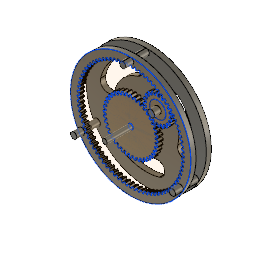
geaarttestv7 (Autodesk Fusion 360 design; units mm, degrees)
description: Spur Gear; Module: 2.025000; Num Teeth: 20; Pressure Angle: 20.000000;
description: Spur Gear; Module: 2.012500; Num Teeth: 40; Pressure Angle: 20.000000;
description: Internal Gear; Module: 2.006300; Num Teeth: 80; Pressure Angle: 20.000000;
Autodesk Fusion 360 part; units mm, degrees
note: some values were not read from the file. Chosen so that the rebuilt part matches the saved one: which face or edge a step refers to. Set by a fixed rule: which sketch regions a step uses.
(part 1 of 7)
sketch "sketch 24727" plane through (0, 0, 0) normal (0, 1, 0) x (1, 0, 0)
  arc A0 (9.2346, -15.5837) -> (8.6942, -15.4391) centre (8.8905, -15.7876) ccw
  spline S0 degree 3 poles (1.6734, -19.8471) (1.7782, -19.3656) (1.7806, -19.0777) (1.7776, -18.982) knots 0 0 0 0 1 1 1 1
  line L0 (3.967, -17.6746) -> (4.1752, -18.6023)
  arc A1 (2.0411, -17.6008) -> (1.6889, -18.0354) centre (2.0872, -17.9981) ccw
  arc A2 (16.6308, -7.1795) -> (16.1086, -7.3802) centre (16.4723, -7.5468) ccw
  arc A3 (20.9592, -7.549) -> (21.3935, -6.2122) centre (0, 0) ccw
  arc A4 (15.4391, -8.6942) -> (16.1086, -7.3802) centre (0, 0) ccw
  spline S1 degree 3 poles (19.3928, -4.5416) (18.9673, -4.2932) (18.6942, -4.2018) (18.6023, -4.1752) knots 0 0 0 0 1 1 1 1
  arc A5 (3.967, -17.6746) -> (3.4977, -17.3701) centre (3.5767, -17.7622) ccw
  arc A6 (-0.7028, -22.2661) -> (0.7028, -22.2661) centre (0, 0) ccw
  arc A7 (18.0354, -1.6889) -> (17.6008, -2.0411) centre (17.9981, -2.0872) ccw
  circle A8 centre (0, 0) radius 12.5
  line L1 (18.0354, -1.6889) -> (18.982, -1.7776)
  arc A9 (7.3802, -16.1086) -> (8.6942, -15.4391) centre (0, 0) ccw
  arc A10 (12.5191, -18.4268) -> (13.6563, -17.6006) centre (0, 0) ccw
  spline S2 degree 3 poles (17.0403, -10.312) (16.7123, -9.9443) (16.4808, -9.773) (16.4016, -9.7193) knots 0 0 0 0 1 1 1 1
  arc A11 (7.3802, -16.1086) -> (7.1795, -16.6308) centre (7.5468, -16.4723) ccw
  spline S3 degree 3 poles (7.7246, -18.3586) (7.6754, -17.8683) (7.5888, -17.5937) (7.5563, -17.5037) knots 0 0 0 0 1 1 1 1
  arc A12 (17.6006, -13.6563) -> (18.4268, -12.5191) centre (0, 0) ccw
  spline S4 degree 3 poles (15.0717, -13.0196) (15.6108, -13.2551) (16.4387, -13.5224) (17.6006, -13.6563) knots 0 0 0 0 1 1 1 1
  arc A13 (15.4391, -8.6942) -> (15.5837, -9.2346) centre (15.7876, -8.8905) ccw
  spline S5 degree 3 poles (21.3935, -6.2122) (20.6023, -5.3509) (19.8994, -4.8382) (19.3928, -4.5416) knots 0 0 0 0 1 1 1 1
  arc A14 (13.5982, -11.9673) -> (13.0396, -11.9968) centre (13.334, -12.2676) ccw
  arc A15 (17.3701, -3.4977) -> (17.6008, -2.0411) centre (0, 0) ccw
  spline S6 degree 3 poles (7.549, -20.9592) (7.7807, -19.8128) (7.7824, -18.9428) (7.7246, -18.3586) knots 0 0 0 0 1 1 1 1
  line L2 (18.6023, -4.1752) -> (17.6746, -3.967)
  arc A16 (17.3701, -3.4977) -> (17.6746, -3.967) centre (17.7622, -3.5767) ccw
  line L3 (1.7776, -18.982) -> (1.6889, -18.0354)
  spline S7 degree 3 poles (0.7028, -22.2661) (1.2774, -21.2475) (1.5478, -20.4206) (1.6734, -19.8471) knots 0 0 0 0 1 1 1 1
  arc A17 (2.0411, -17.6008) -> (3.4977, -17.3701) centre (0, 0) ccw
  line L4 (7.5563, -17.5037) -> (7.1795, -16.6308)
  spline S8 degree 3 poles (13.0197, -15.073) (12.8214, -14.6219) (12.6541, -14.3875) (12.5955, -14.312) knots 0 0 0 0 1 1 1 1
  line L5 (9.2346, -15.5837) -> (9.7193, -16.4016)
  line L6 (16.4016, -9.7193) -> (15.5837, -9.2346)
  line L7 (12.5955, -14.312) -> (11.9673, -13.5982)
  arc A18 (11.9968, -13.0396) -> (11.9673, -13.5982) centre (12.2676, -13.334) ccw
  spline S9 degree 3 poles (13.6563, -17.6006) (13.5224, -16.4387) (13.2551, -15.6108) (13.0197, -15.073) knots 0 0 0 0 1 1 1 1
  spline S10 degree 3 poles (10.3107, -17.0398) (10.7507, -17.4304) (11.4555, -17.9404) (12.5191, -18.4268) knots 0 0 0 0 1 1 1 1
  spline S11 degree 3 poles (9.7193, -16.4016) (9.773, -16.4808) (9.9443, -16.7123) (10.3107, -17.0398) knots 0 0 0 0 1 1 1 1
  arc A19 (11.9968, -13.0396) -> (13.0396, -11.9968) centre (0, 0) ccw
  line L8 (13.5982, -11.9673) -> (14.312, -12.5955)
  spline S12 degree 3 poles (18.3573, -7.725) (18.9428, -7.7824) (19.8128, -7.7807) (20.9592, -7.549) knots 0 0 0 0 1 1 1 1
  spline S13 degree 3 poles (18.4268, -12.5191) (17.9404, -11.4555) (17.4304, -10.7507) (17.0403, -10.312) knots 0 0 0 0 1 1 1 1
  line L9 (16.6308, -7.1795) -> (17.5037, -7.5563)
  spline S14 degree 3 poles (17.5037, -7.5563) (17.5937, -7.5888) (17.8683, -7.6754) (18.3573, -7.725) knots 0 0 0 0 1 1 1 1
  spline S15 degree 3 poles (4.5405, -19.392) (4.8382, -19.8994) (5.3509, -20.6023) (6.2122, -21.3935) knots 0 0 0 0 1 1 1 1
  spline S16 degree 3 poles (14.312, -12.5955) (14.3875, -12.6541) (14.6219, -12.8214) (15.0717, -13.0196) knots 0 0 0 0 1 1 1 1
  arc A20 (6.2122, -21.3935) -> (7.549, -20.9592) centre (0, 0) ccw
  spline S17 degree 3 poles (4.1752, -18.6023) (4.2018, -18.6942) (4.2932, -18.9673) (4.5405, -19.392) knots 0 0 0 0 1 1 1 1
  spline S18 degree 3 poles (-1.6742, -19.846) (-1.5478, -20.4206) (-1.2774, -21.2475) (-0.7028, -22.2661) knots 0 0 0 0 1 1 1 1
  spline S19 degree 3 poles (-1.7776, -18.982) (-1.7806, -19.0777) (-1.7782, -19.3656) (-1.6742, -19.846) knots 0 0 0 0 1 1 1 1
  line L10 (15.5837, 9.2346) -> (16.4016, 9.7193)
  arc A21 (15.5837, 9.2346) -> (15.4391, 8.6942) centre (15.7876, 8.8905) ccw
  spline S20 degree 3 poles (18.3586, 7.7246) (17.8683, 7.6754) (17.5937, 7.5888) (17.5037, 7.5563) knots 0 0 0 0 1 1 1 1
  line L11 (14.312, 12.5955) -> (13.5982, 11.9673)
  spline S21 degree 3 poles (19.8471, 1.6734) (19.3656, 1.7782) (19.0777, 1.7806) (18.982, 1.7776) knots 0 0 0 0 1 1 1 1
  arc A22 (21.3935, 6.2122) -> (20.9592, 7.549) centre (0, 0) ccw
  line L12 (17.5037, 7.5563) -> (16.6308, 7.1795)
  line L13 (11.9673, 13.5982) -> (12.5955, 14.312)
  spline S22 degree 3 poles (15.073, 13.0197) (14.6219, 12.8214) (14.3875, 12.6541) (14.312, 12.5955) knots 0 0 0 0 1 1 1 1
  arc A23 (11.9673, 13.5982) -> (11.9968, 13.0396) centre (12.2676, 13.334) ccw
  arc A24 (13.0396, 11.9968) -> (13.5982, 11.9673) centre (13.334, 12.2676) ccw
  arc A25 (13.0396, 11.9968) -> (11.9968, 13.0396) centre (0, 0) ccw
  spline S23 degree 3 poles (13.0196, 15.0717) (13.2551, 15.6108) (13.5224, 16.4387) (13.6563, 17.6006) knots 0 0 0 0 1 1 1 1
  spline S24 degree 3 poles (18.982, -1.7776) (19.0777, -1.7806) (19.3656, -1.7782) (19.846, -1.6742) knots 0 0 0 0 1 1 1 1
  spline S25 degree 3 poles (12.5955, 14.312) (12.6541, 14.3875) (12.8214, 14.6219) (13.0196, 15.0717) knots 0 0 0 0 1 1 1 1
  arc A26 (17.6746, 3.967) -> (17.3701, 3.4977) centre (17.7622, 3.5767) ccw
  spline S26 degree 3 poles (19.392, 4.5405) (19.8994, 4.8382) (20.6023, 5.3509) (21.3935, 6.2122) knots 0 0 0 0 1 1 1 1
  arc A27 (16.1086, 7.3802) -> (15.4391, 8.6942) centre (0, 0) ccw
  line L14 (18.982, 1.7776) -> (18.0354, 1.6889)
  arc A28 (17.6008, 2.0411) -> (17.3701, 3.4977) centre (0, 0) ccw
  arc A29 (22.2661, -0.7028) -> (22.2661, 0.7028) centre (0, 0) ccw
  spline S27 degree 3 poles (19.846, -1.6742) (20.4206, -1.5478) (21.2475, -1.2774) (22.2661, -0.7028) knots 0 0 0 0 1 1 1 1
  spline S28 degree 3 poles (22.2661, 0.7028) (21.2475, 1.2774) (20.4206, 1.5478) (19.8471, 1.6734) knots 0 0 0 0 1 1 1 1
  arc A30 (17.6008, 2.0411) -> (18.0354, 1.6889) centre (17.9981, 2.0872) ccw
  line L15 (17.6746, 3.967) -> (18.6023, 4.1752)
  spline S29 degree 3 poles (20.9592, 7.549) (19.8128, 7.7807) (18.9428, 7.7824) (18.3586, 7.7246) knots 0 0 0 0 1 1 1 1
  spline S30 degree 3 poles (18.6023, 4.1752) (18.6942, 4.2018) (18.9673, 4.2932) (19.392, 4.5405) knots 0 0 0 0 1 1 1 1
  spline S31 degree 3 poles (16.4016, 9.7193) (16.4808, 9.773) (16.7123, 9.9443) (17.0398, 10.3107) knots 0 0 0 0 1 1 1 1
  arc A31 (18.4268, 12.5191) -> (17.6006, 13.6563) centre (0, 0) ccw
  spline S32 degree 3 poles (17.6006, 13.6563) (16.4387, 13.5224) (15.6108, 13.2551) (15.073, 13.0197) knots 0 0 0 0 1 1 1 1
  spline S33 degree 3 poles (17.0398, 10.3107) (17.4304, 10.7507) (17.9404, 11.4555) (18.4268, 12.5191) knots 0 0 0 0 1 1 1 1
  arc A32 (16.1086, 7.3802) -> (16.6308, 7.1795) centre (16.4723, 7.5468) ccw
  spline S34 degree 3 poles (1.6742, 19.846) (1.5478, 20.4206) (1.2774, 21.2475) (0.7028, 22.2661) knots 0 0 0 0 1 1 1 1
  spline S35 degree 3 poles (1.7776, 18.982) (1.7806, 19.0777) (1.7782, 19.3656) (1.6742, 19.846) knots 0 0 0 0 1 1 1 1
  line L16 (-7.5563, 17.5037) -> (-7.1795, 16.6308)
  spline S36 degree 3 poles (-15.0717, 13.0196) (-15.6108, 13.2551) (-16.4387, 13.5224) (-17.6006, 13.6563) knots 0 0 0 0 1 1 1 1
  arc A33 (-6.2122, 21.3935) -> (-7.549, 20.9592) centre (0, 0) ccw
  arc A34 (-3.967, 17.6746) -> (-3.4977, 17.3701) centre (-3.5767, 17.7622) ccw
  arc A35 (3.4977, 17.3701) -> (3.967, 17.6746) centre (3.5767, 17.7622) ccw
  spline S37 degree 3 poles (-4.5405, 19.392) (-4.8382, 19.8994) (-5.3509, 20.6023) (-6.2122, 21.3935) knots 0 0 0 0 1 1 1 1
  arc A36 (-13.5982, 11.9673) -> (-13.0396, 11.9968) centre (-13.334, 12.2676) ccw
  arc A37 (-15.4391, 8.6942) -> (-15.5837, 9.2346) centre (-15.7876, 8.8905) ccw
  arc A38 (8.6942, 15.4391) -> (7.3802, 16.1086) centre (0, 0) ccw
  spline S38 degree 3 poles (-17.0403, 10.312) (-16.7123, 9.9443) (-16.4808, 9.773) (-16.4016, 9.7193) knots 0 0 0 0 1 1 1 1
  spline S39 degree 3 poles (-13.0197, 15.073) (-12.8214, 14.6219) (-12.6541, 14.3875) (-12.5955, 14.312) knots 0 0 0 0 1 1 1 1
  spline S40 degree 3 poles (-1.6734, 19.8471) (-1.7782, 19.3656) (-1.7806, 19.0777) (-1.7776, 18.982) knots 0 0 0 0 1 1 1 1
  spline S41 degree 3 poles (-9.7193, 16.4016) (-9.773, 16.4808) (-9.9443, 16.7123) (-10.3107, 17.0398) knots 0 0 0 0 1 1 1 1
  spline S42 degree 3 poles (-14.312, 12.5955) (-14.3875, 12.6541) (-14.6219, 12.8214) (-15.0717, 13.0196) knots 0 0 0 0 1 1 1 1
  spline S43 degree 3 poles (-18.4268, 12.5191) (-17.9404, 11.4555) (-17.4304, 10.7507) (-17.0403, 10.312) knots 0 0 0 0 1 1 1 1
  line L17 (9.7193, 16.4016) -> (9.2346, 15.5837)
  line L18 (-12.5955, 14.312) -> (-11.9673, 13.5982)
  arc A39 (-2.0411, 17.6008) -> (-1.6889, 18.0354) centre (-2.0872, 17.9981) ccw
  arc A40 (1.6889, 18.0354) -> (2.0411, 17.6008) centre (2.0872, 17.9981) ccw
  spline S44 degree 3 poles (-7.7246, 18.3586) (-7.6754, 17.8683) (-7.5888, 17.5937) (-7.5563, 17.5037) knots 0 0 0 0 1 1 1 1
  spline S45 degree 3 poles (-4.1752, 18.6023) (-4.2018, 18.6942) (-4.2932, 18.9673) (-4.5405, 19.392) knots 0 0 0 0 1 1 1 1
  arc A41 (7.549, 20.9592) -> (6.2122, 21.3935) centre (0, 0) ccw
  arc A42 (13.6563, 17.6006) -> (12.5191, 18.4268) centre (0, 0) ccw
  arc A43 (8.6942, 15.4391) -> (9.2346, 15.5837) centre (8.8905, 15.7876) ccw
  arc A44 (3.4977, 17.3701) -> (2.0411, 17.6008) centre (0, 0) ccw
  spline S46 degree 3 poles (-7.549, 20.9592) (-7.7807, 19.8128) (-7.7824, 18.9428) (-7.7246, 18.3586) knots 0 0 0 0 1 1 1 1
  spline S47 degree 3 poles (10.312, 17.0403) (9.9443, 16.7123) (9.773, 16.4808) (9.7193, 16.4016) knots 0 0 0 0 1 1 1 1
  arc A45 (-9.2346, 15.5837) -> (-8.6942, 15.4391) centre (-8.8905, 15.7876) ccw
  spline S48 degree 3 poles (6.2122, 21.3935) (5.3509, 20.6023) (4.8382, 19.8994) (4.5416, 19.3928) knots 0 0 0 0 1 1 1 1
  line L19 (4.1752, 18.6023) -> (3.967, 17.6746)
  spline S49 degree 3 poles (12.5191, 18.4268) (11.4555, 17.9404) (10.7507, 17.4304) (10.312, 17.0403) knots 0 0 0 0 1 1 1 1
  spline S50 degree 3 poles (-0.7028, 22.2661) (-1.2774, 21.2475) (-1.5478, 20.4206) (-1.6734, 19.8471) knots 0 0 0 0 1 1 1 1
  line L20 (-3.967, 17.6746) -> (-4.1752, 18.6023)
  arc A46 (-7.3802, 16.1086) -> (-7.1795, 16.6308) centre (-7.5468, 16.4723) ccw
  arc A47 (-12.5191, 18.4268) -> (-13.6563, 17.6006) centre (0, 0) ccw
  spline S51 degree 3 poles (7.5563, 17.5037) (7.5888, 17.5937) (7.6754, 17.8683) (7.725, 18.3573) knots 0 0 0 0 1 1 1 1
  line L21 (-1.7776, 18.982) -> (-1.6889, 18.0354)
  spline S52 degree 3 poles (-10.3107, 17.0398) (-10.7507, 17.4304) (-11.4555, 17.9404) (-12.5191, 18.4268) knots 0 0 0 0 1 1 1 1
  arc A48 (7.1795, 16.6308) -> (7.3802, 16.1086) centre (7.5468, 16.4723) ccw
  arc A49 (-2.0411, 17.6008) -> (-3.4977, 17.3701) centre (0, 0) ccw
  line L22 (-9.2346, 15.5837) -> (-9.7193, 16.4016)
  spline S53 degree 3 poles (4.5416, 19.3928) (4.2932, 18.9673) (4.2018, 18.6942) (4.1752, 18.6023) knots 0 0 0 0 1 1 1 1
  spline S54 degree 3 poles (-13.6563, 17.6006) (-13.5224, 16.4387) (-13.2551, 15.6108) (-13.0197, 15.073) knots 0 0 0 0 1 1 1 1
  spline S55 degree 3 poles (7.725, 18.3573) (7.7824, 18.9428) (7.7807, 19.8128) (7.549, 20.9592) knots 0 0 0 0 1 1 1 1
  line L23 (7.1795, 16.6308) -> (7.5563, 17.5037)
  arc A50 (0.7028, 22.2661) -> (-0.7028, 22.2661) centre (0, 0) ccw
  arc A51 (-17.6006, 13.6563) -> (-18.4268, 12.5191) centre (0, 0) ccw
  arc A52 (-11.9968, 13.0396) -> (-11.9673, 13.5982) centre (-12.2676, 13.334) ccw
  line L24 (-13.5982, 11.9673) -> (-14.312, 12.5955)
  arc A53 (-7.3802, 16.1086) -> (-8.6942, 15.4391) centre (0, 0) ccw
  arc A54 (-11.9968, 13.0396) -> (-13.0396, 11.9968) centre (0, 0) ccw
  line L25 (1.6889, 18.0354) -> (1.7776, 18.982)
  arc A55 (-15.4391, 8.6942) -> (-16.1086, 7.3802) centre (0, 0) ccw
  line L26 (-17.5037, -7.5563) -> (-16.6308, -7.1795)
  line L27 (-9.7193, -16.4016) -> (-9.2346, -15.5837)
  arc A56 (-8.6942, -15.4391) -> (-9.2346, -15.5837) centre (-8.8905, -15.7876) ccw
  spline S56 degree 3 poles (-17.0398, -10.3107) (-17.4304, -10.7507) (-17.9404, -11.4555) (-18.4268, -12.5191) knots 0 0 0 0 1 1 1 1
  spline S57 degree 3 poles (-6.2122, -21.3935) (-5.3509, -20.6023) (-4.8382, -19.8994) (-4.5416, -19.3928) knots 0 0 0 0 1 1 1 1
  line L28 (-1.6889, -18.0354) -> (-1.7776, -18.982)
  arc A57 (-17.3701, 3.4977) -> (-17.6008, 2.0411) centre (0, 0) ccw
  line L29 (-18.982, -1.7776) -> (-18.0354, -1.6889)
  spline S58 degree 3 poles (-18.3573, 7.725) (-18.9428, 7.7824) (-19.8128, 7.7807) (-20.9592, 7.549) knots 0 0 0 0 1 1 1 1
  arc A58 (-16.6308, 7.1795) -> (-16.1086, 7.3802) centre (-16.4723, 7.5468) ccw
  spline S59 degree 3 poles (-18.982, 1.7776) (-19.0777, 1.7806) (-19.3656, 1.7782) (-19.846, 1.6742) knots 0 0 0 0 1 1 1 1
  spline S60 degree 3 poles (-13.0196, -15.0717) (-13.2551, -15.6108) (-13.5224, -16.4387) (-13.6563, -17.6006) knots 0 0 0 0 1 1 1 1
  spline S61 degree 3 poles (-17.5037, 7.5563) (-17.5937, 7.5888) (-17.8683, 7.6754) (-18.3573, 7.725) knots 0 0 0 0 1 1 1 1
  arc A59 (-17.6746, -3.967) -> (-17.3701, -3.4977) centre (-17.7622, -3.5767) ccw
  spline S62 degree 3 poles (-20.9592, -7.549) (-19.8128, -7.7807) (-18.9428, -7.7824) (-18.3586, -7.7246) knots 0 0 0 0 1 1 1 1
  line L30 (-16.4016, 9.7193) -> (-15.5837, 9.2346)
  line L31 (-16.6308, 7.1795) -> (-17.5037, 7.5563)
  arc A60 (-17.6008, -2.0411) -> (-18.0354, -1.6889) centre (-17.9981, -2.0872) ccw
  line L32 (-18.6023, 4.1752) -> (-17.6746, 3.967)
  arc A61 (-16.1086, -7.3802) -> (-16.6308, -7.1795) centre (-16.4723, -7.5468) ccw
  line L33 (-15.5837, -9.2346) -> (-16.4016, -9.7193)
  spline S63 degree 3 poles (-19.3928, 4.5416) (-18.9673, 4.2932) (-18.6942, 4.2018) (-18.6023, 4.1752) knots 0 0 0 0 1 1 1 1
  arc A62 (-18.4268, -12.5191) -> (-17.6006, -13.6563) centre (0, 0) ccw
  spline S64 degree 3 poles (-18.3586, -7.7246) (-17.8683, -7.6754) (-17.5937, -7.5888) (-17.5037, -7.5563) knots 0 0 0 0 1 1 1 1
  arc A63 (-13.0396, -11.9968) -> (-11.9968, -13.0396) centre (0, 0) ccw
  line L34 (-11.9673, -13.5982) -> (-12.5955, -14.312)
  arc A64 (-22.2661, 0.7028) -> (-22.2661, -0.7028) centre (0, 0) ccw
  spline S65 degree 3 poles (-17.6006, -13.6563) (-16.4387, -13.5224) (-15.6108, -13.2551) (-15.073, -13.0197) knots 0 0 0 0 1 1 1 1
  spline S66 degree 3 poles (-15.073, -13.0197) (-14.6219, -12.8214) (-14.3875, -12.6541) (-14.312, -12.5955) knots 0 0 0 0 1 1 1 1
  arc A65 (-13.0396, -11.9968) -> (-13.5982, -11.9673) centre (-13.334, -12.2676) ccw
  spline S67 degree 3 poles (-16.4016, -9.7193) (-16.4808, -9.773) (-16.7123, -9.9443) (-17.0398, -10.3107) knots 0 0 0 0 1 1 1 1
  arc A66 (-13.6563, -17.6006) -> (-12.5191, -18.4268) centre (0, 0) ccw
  spline S68 degree 3 poles (-18.6023, -4.1752) (-18.6942, -4.2018) (-18.9673, -4.2932) (-19.392, -4.5405) knots 0 0 0 0 1 1 1 1
  spline S69 degree 3 poles (-22.2661, -0.7028) (-21.2475, -1.2774) (-20.4206, -1.5478) (-19.8471, -1.6734) knots 0 0 0 0 1 1 1 1
  arc A67 (-18.0354, 1.6889) -> (-17.6008, 2.0411) centre (-17.9981, 2.0872) ccw
  arc A68 (-17.3701, 3.4977) -> (-17.6746, 3.967) centre (-17.7622, 3.5767) ccw
  spline S70 degree 3 poles (-21.3935, 6.2122) (-20.6023, 5.3509) (-19.8994, 4.8382) (-19.3928, 4.5416) knots 0 0 0 0 1 1 1 1
  spline S71 degree 3 poles (-19.392, -4.5405) (-19.8994, -4.8382) (-20.6023, -5.3509) (-21.3935, -6.2122) knots 0 0 0 0 1 1 1 1
  arc A69 (-21.3935, -6.2122) -> (-20.9592, -7.549) centre (0, 0) ccw
  arc A70 (-15.5837, -9.2346) -> (-15.4391, -8.6942) centre (-15.7876, -8.8905) ccw
  arc A71 (-17.6008, -2.0411) -> (-17.3701, -3.4977) centre (0, 0) ccw
  line L35 (-17.6746, -3.967) -> (-18.6023, -4.1752)
  arc A72 (-11.9673, -13.5982) -> (-11.9968, -13.0396) centre (-12.2676, -13.334) ccw
  spline S72 degree 3 poles (-10.312, -17.0403) (-9.9443, -16.7123) (-9.773, -16.4808) (-9.7193, -16.4016) knots 0 0 0 0 1 1 1 1
  arc A73 (-20.9592, 7.549) -> (-21.3935, 6.2122) centre (0, 0) ccw
  arc A74 (-8.6942, -15.4391) -> (-7.3802, -16.1086) centre (0, 0) ccw
  spline S73 degree 3 poles (-12.5191, -18.4268) (-11.4555, -17.9404) (-10.7507, -17.4304) (-10.312, -17.0403) knots 0 0 0 0 1 1 1 1
  spline S74 degree 3 poles (-12.5955, -14.312) (-12.6541, -14.3875) (-12.8214, -14.6219) (-13.0196, -15.0717) knots 0 0 0 0 1 1 1 1
  spline S75 degree 3 poles (-19.846, 1.6742) (-20.4206, 1.5478) (-21.2475, 1.2774) (-22.2661, 0.7028) knots 0 0 0 0 1 1 1 1
  line L36 (-7.1795, -16.6308) -> (-7.5563, -17.5037)
  spline S76 degree 3 poles (-7.5563, -17.5037) (-7.5888, -17.5937) (-7.6754, -17.8683) (-7.725, -18.3573) knots 0 0 0 0 1 1 1 1
  arc A75 (-7.1795, -16.6308) -> (-7.3802, -16.1086) centre (-7.5468, -16.4723) ccw
  spline S77 degree 3 poles (-7.725, -18.3573) (-7.7824, -18.9428) (-7.7807, -19.8128) (-7.549, -20.9592) knots 0 0 0 0 1 1 1 1
  arc A76 (-16.1086, -7.3802) -> (-15.4391, -8.6942) centre (0, 0) ccw
  arc A77 (-7.549, -20.9592) -> (-6.2122, -21.3935) centre (0, 0) ccw
  line L37 (-18.0354, 1.6889) -> (-18.982, 1.7776)
  spline S78 degree 3 poles (-19.8471, -1.6734) (-19.3656, -1.7782) (-19.0777, -1.7806) (-18.982, -1.7776) knots 0 0 0 0 1 1 1 1
  line L38 (-14.312, -12.5955) -> (-13.5982, -11.9673)
  line L39 (-4.1752, -18.6023) -> (-3.967, -17.6746)
  arc A78 (-1.6889, -18.0354) -> (-2.0411, -17.6008) centre (-2.0872, -17.9981) ccw
  arc A79 (-3.4977, -17.3701) -> (-2.0411, -17.6008) centre (0, 0) ccw
  arc A80 (-3.4977, -17.3701) -> (-3.967, -17.6746) centre (-3.5767, -17.7622) ccw
  spline S79 degree 3 poles (-4.5416, -19.3928) (-4.2932, -18.9673) (-4.2018, -18.6942) (-4.1752, -18.6023) knots 0 0 0 0 1 1 1 1
extrude "Extrude1" add sketch "sketch 24727" along normal blind 8 makes body 1 in component "Spur Gear (20 teeth)"
sketch "Sketch1" plane through (0, 0, 0) normal (0, 1, 0) x (1, 0, 0) in component "Spur Gear (20 teeth)"
  circle A0 centre (0, 0) radius 20.25 construction
sketch "sketch 26269" plane through (0, 0, 0) normal (0, 1, 0) x (1, 0, 0)
  spline S0 degree 3 poles (-13.6938, -35.5383) (-13.7432, -35.732) (-13.808, -36.0399) (-13.8582, -36.4722) knots 0 0 0 0 1 1 1 1
  spline S1 degree 3 poles (-24.2197, -34.6367) (-22.8543, -33.8927) (-21.9375, -33.1795) (-21.3609, -32.6493) knots 0 0 0 0 1 1 1 1
  spline S2 degree 3 poles (-18.5031, -37.999) (-17.271, -37.0506) (-16.477, -36.2028) (-15.9905, -35.5889) knots 0 0 0 0 1 1 1 1
  arc A0 (-20.1803, -31.8848) -> (-19.2479, -32.4562) centre (0, 0) ccw
  arc A1 (-14.944, -34.6491) -> (-13.9336, -35.0676) centre (0, 0) ccw
  arc A2 (-14.944, -34.6491) -> (-15.4464, -34.8123) centre (-15.1024, -35.0164) ccw
  spline S3 degree 3 poles (-15.9905, -35.5889) (-15.7204, -35.2478) (-15.5484, -34.9843) (-15.4464, -34.8123) knots 0 0 0 0 1 1 1 1
  arc A3 (-13.6938, -35.5383) -> (-13.9336, -35.0676) centre (-14.0813, -35.4393) ccw
  arc A4 (-13.7857, -39.953) -> (-12.331, -40.4257) centre (0, 0) ccw
  spline S4 degree 3 poles (-19.0846, -32.9586) (-19.1638, -33.1422) (-19.2759, -33.4362) (-19.3931, -33.8552) knots 0 0 0 0 1 1 1 1
  spline S5 degree 3 poles (-12.331, -40.4257) (-11.2623, -39.2962) (-10.6107, -38.3346) (-10.2263, -37.6523) knots 0 0 0 0 1 1 1 1
  spline S6 degree 3 poles (-21.3609, -32.6493) (-21.0408, -32.3546) (-20.8297, -32.1213) (-20.7021, -31.9674) knots 0 0 0 0 1 1 1 1
  arc A5 (-20.1803, -31.8848) -> (-20.7021, -31.9674) centre (-20.3942, -32.2228) ccw
  arc A6 (-19.866, -37.3046) -> (-18.5031, -37.999) centre (0, 0) ccw
  spline S7 degree 3 poles (-19.3931, -33.8552) (-19.6037, -34.6096) (-19.823, -35.7503) (-19.866, -37.3046) knots 0 0 0 0 1 1 1 1
  spline S8 degree 3 poles (-7.9658, -37.243) (-7.9843, -37.442) (-8.0001, -37.7562) (-7.9821, -38.191) knots 0 0 0 0 1 1 1 1
  arc A7 (-7.9658, -37.243) -> (-8.2763, -36.8156) centre (-8.364, -37.2058) ccw
  arc A8 (-9.3397, -36.5603) -> (-8.2763, -36.8156) centre (0, 0) ccw
  arc A9 (-9.3397, -36.5603) -> (-9.8104, -36.8001) centre (-9.4387, -36.9478) ccw
  spline S9 degree 3 poles (-13.8582, -36.4722) (-13.9482, -37.2502) (-13.9863, -38.4112) (-13.7857, -39.953) knots 0 0 0 0 1 1 1 1
  spline S10 degree 3 poles (-10.2263, -37.6523) (-10.0128, -37.273) (-9.8842, -36.9859) (-9.8104, -36.8001) knots 0 0 0 0 1 1 1 1
  spline S11 degree 3 poles (-5.8552, -41.857) (-4.9764, -40.5743) (-4.4833, -39.5225) (-4.2102, -38.7884) knots 0 0 0 0 1 1 1 1
  arc A10 (-3.5054, -37.5712) -> (-2.4152, -37.657) centre (0, 0) ccw
  arc A11 (-3.5054, -37.5712) -> (-3.9328, -37.8817) centre (-3.5426, -37.9695) ccw
  spline S12 degree 3 poles (-1.9094, -38.9695) (-1.7546, -39.7373) (-1.4321, -40.8532) (-0.7648, -42.2576) knots 0 0 0 0 1 1 1 1
  arc A12 (-0.7648, -42.2576) -> (0.7648, -42.2576) centre (0, 0) ccw
  spline S13 degree 3 poles (-4.2102, -38.7884) (-4.0588, -38.3805) (-3.9767, -38.0767) (-3.9328, -37.8817) knots 0 0 0 0 1 1 1 1
  arc A13 (-7.3659, -41.6177) -> (-5.8552, -41.857) centre (0, 0) ccw
  spline S14 degree 3 poles (-7.9821, -38.191) (-7.9493, -38.9736) (-7.8053, -40.1262) (-7.3659, -41.6177) knots 0 0 0 0 1 1 1 1
  spline S15 degree 3 poles (4.2102, -38.7884) (4.4833, -39.5225) (4.9764, -40.5743) (5.8552, -41.857) knots 0 0 0 0 1 1 1 1
  spline S16 degree 3 poles (0.7648, -42.2576) (1.4321, -40.8532) (1.7546, -39.7373) (1.9094, -38.9695) knots 0 0 0 0 1 1 1 1
  spline S17 degree 3 poles (1.9094, -38.9695) (1.9952, -38.5429) (2.0288, -38.23) (2.0416, -38.0306) knots 0 0 0 0 1 1 1 1
  spline S18 degree 3 poles (3.9328, -37.8817) (3.9767, -38.0767) (4.0588, -38.3805) (4.2102, -38.7884) knots 0 0 0 0 1 1 1 1
  spline S19 degree 3 poles (-2.0416, -38.0306) (-2.0288, -38.23) (-1.9952, -38.5429) (-1.9094, -38.9695) knots 0 0 0 0 1 1 1 1
  arc A14 (-2.0416, -38.0306) -> (-2.4152, -37.657) centre (-2.4408, -38.0562) ccw
  arc A15 (2.4152, -37.657) -> (2.0416, -38.0306) centre (2.4408, -38.0562) ccw
  arc A16 (2.4152, -37.657) -> (3.5054, -37.5712) centre (0, 0) ccw
  arc A17 (3.9328, -37.8817) -> (3.5054, -37.5712) centre (3.5426, -37.9695) ccw
  arc A18 (5.8552, -41.857) -> (7.3659, -41.6177) centre (0, 0) ccw
  circle A19 centre (0, 0) radius 3.85
  arc A20 (31.8848, -20.1803) -> (32.4562, -19.2479) centre (0, 0) ccw
  arc A21 (37.5712, -3.5054) -> (37.8817, -3.9328) centre (37.9695, -3.5426) ccw
  spline S20 degree 3 poles (41.857, -5.8552) (40.5743, -4.9764) (39.5225, -4.4833) (38.7884, -4.2102) knots 0 0 0 0 1 1 1 1
  arc A22 (37.5712, -3.5054) -> (37.657, -2.4152) centre (0, 0) ccw
  spline S21 degree 3 poles (38.7884, -4.2102) (38.3805, -4.0588) (38.0767, -3.9767) (37.8817, -3.9328) knots 0 0 0 0 1 1 1 1
  spline S22 degree 3 poles (32.6493, -21.3609) (32.3546, -21.0408) (32.1213, -20.8297) (31.9674, -20.7021) knots 0 0 0 0 1 1 1 1
  arc A23 (31.8848, -20.1803) -> (31.9674, -20.7021) centre (32.2228, -20.3942) ccw
  spline S23 degree 3 poles (34.6367, -24.2197) (33.8927, -22.8543) (33.1795, -21.9375) (32.6493, -21.3609) knots 0 0 0 0 1 1 1 1
  arc A24 (37.3046, -19.866) -> (37.999, -18.5031) centre (0, 0) ccw
  arc A25 (34.6491, -14.944) -> (35.0676, -13.9336) centre (0, 0) ccw
  arc A26 (32.9586, -19.0846) -> (32.4562, -19.2479) centre (32.8002, -19.4519) ccw
  spline S24 degree 3 poles (32.9586, -19.0846) (33.1422, -19.1638) (33.4362, -19.2759) (33.8552, -19.3931) knots 0 0 0 0 1 1 1 1
  spline S25 degree 3 poles (33.8552, -19.3931) (34.6096, -19.6037) (35.7503, -19.823) (37.3046, -19.866) knots 0 0 0 0 1 1 1 1
  spline S26 degree 3 poles (37.999, -18.5031) (37.0506, -17.271) (36.2028, -16.477) (35.5889, -15.9905) knots 0 0 0 0 1 1 1 1
  arc A27 (34.6491, -14.944) -> (34.8123, -15.4464) centre (35.0164, -15.1024) ccw
  arc A28 (36.5603, -9.3397) -> (36.8001, -9.8104) centre (36.9478, -9.4387) ccw
  spline S27 degree 3 poles (35.5889, -15.9905) (35.2478, -15.7204) (34.9843, -15.5484) (34.8123, -15.4464) knots 0 0 0 0 1 1 1 1
  spline S28 degree 3 poles (35.5383, -13.6938) (35.732, -13.7432) (36.0399, -13.808) (36.4722, -13.8582) knots 0 0 0 0 1 1 1 1
  arc A29 (37.243, -7.9658) -> (36.8156, -8.2763) centre (37.2058, -8.364) ccw
  spline S29 degree 3 poles (36.4722, -13.8582) (37.2502, -13.9482) (38.4112, -13.9863) (39.953, -13.7857) knots 0 0 0 0 1 1 1 1
  arc A30 (39.953, -13.7857) -> (40.4257, -12.331) centre (0, 0) ccw
  arc A31 (36.5603, -9.3397) -> (36.8156, -8.2763) centre (0, 0) ccw
  spline S30 degree 3 poles (37.6523, -10.2263) (37.273, -10.0128) (36.9859, -9.8842) (36.8001, -9.8104) knots 0 0 0 0 1 1 1 1
  arc A32 (35.5383, -13.6938) -> (35.0676, -13.9336) centre (35.4393, -14.0813) ccw
  spline S31 degree 3 poles (40.4257, -12.331) (39.2962, -11.2623) (38.3346, -10.6107) (37.6523, -10.2263) knots 0 0 0 0 1 1 1 1
  spline S32 degree 3 poles (37.243, -7.9658) (37.442, -7.9843) (37.7562, -8.0001) (38.191, -7.9821) knots 0 0 0 0 1 1 1 1
  spline S33 degree 3 poles (-38.0306, 2.0416) (-38.23, 2.0288) (-38.5429, 1.9952) (-38.9695, 1.9094) knots 0 0 0 0 1 1 1 1
  arc A33 (-37.5712, 3.5054) -> (-37.8817, 3.9328) centre (-37.9695, 3.5426) ccw
  arc A34 (-37.5712, 3.5054) -> (-37.657, 2.4152) centre (0, 0) ccw
  arc A35 (41.6177, -7.3659) -> (41.857, -5.8552) centre (0, 0) ccw
  spline S34 degree 3 poles (38.191, -7.9821) (38.9736, -7.9493) (40.1262, -7.8053) (41.6177, -7.3659) knots 0 0 0 0 1 1 1 1
  arc A36 (-38.0306, 2.0416) -> (-37.657, 2.4152) centre (-38.0562, 2.4408) ccw
  spline S35 degree 3 poles (-38.7884, 4.2102) (-38.3805, 4.0588) (-38.0767, 3.9767) (-37.8817, 3.9328) knots 0 0 0 0 1 1 1 1
  spline S36 degree 3 poles (-38.9695, -1.9094) (-38.5429, -1.9952) (-38.23, -2.0288) (-38.0306, -2.0416) knots 0 0 0 0 1 1 1 1
  arc A37 (-37.657, -2.4152) -> (-38.0306, -2.0416) centre (-38.0562, -2.4408) ccw
  arc A38 (-42.2576, 0.7648) -> (-42.2576, -0.7648) centre (0, 0) ccw
  arc A39 (-37.657, -2.4152) -> (-37.5712, -3.5054) centre (0, 0) ccw
  arc A40 (-37.8817, -3.9328) -> (-37.5712, -3.5054) centre (-37.9695, -3.5426) ccw
  spline S37 degree 3 poles (-38.9695, 1.9094) (-39.7373, 1.7546) (-40.8532, 1.4321) (-42.2576, 0.7648) knots 0 0 0 0 1 1 1 1
  spline S38 degree 3 poles (-42.2576, -0.7648) (-40.8532, -1.4321) (-39.7373, -1.7546) (-38.9695, -1.9094) knots 0 0 0 0 1 1 1 1
  spline S39 degree 3 poles (-37.8817, -3.9328) (-38.0767, -3.9767) (-38.3805, -4.0588) (-38.7884, -4.2102) knots 0 0 0 0 1 1 1 1
  spline S40 degree 3 poles (-38.7884, -4.2102) (-39.5225, -4.4833) (-40.5743, -4.9764) (-41.857, -5.8552) knots 0 0 0 0 1 1 1 1
  arc A41 (-41.857, -5.8552) -> (-41.6177, -7.3659) centre (0, 0) ccw
  spline S41 degree 3 poles (-38.191, -7.9821) (-37.7562, -8.0001) (-37.442, -7.9843) (-37.243, -7.9658) knots 0 0 0 0 1 1 1 1
  arc A42 (-36.8001, -9.8104) -> (-36.5603, -9.3397) centre (-36.9478, -9.4387) ccw
  arc A43 (-36.8156, -8.2763) -> (-37.243, -7.9658) centre (-37.2058, -8.364) ccw
  arc A44 (-36.8156, -8.2763) -> (-36.5603, -9.3397) centre (0, 0) ccw
  spline S42 degree 3 poles (-41.6177, -7.3659) (-40.1262, -7.8053) (-38.9736, -7.9493) (-38.191, -7.9821) knots 0 0 0 0 1 1 1 1
  arc A45 (-40.4257, -12.331) -> (-39.953, -13.7857) centre (0, 0) ccw
  spline S43 degree 3 poles (-36.8001, -9.8104) (-36.9859, -9.8842) (-37.273, -10.0128) (-37.6523, -10.2263) knots 0 0 0 0 1 1 1 1
  spline S44 degree 3 poles (-36.4722, -13.8582) (-36.0399, -13.808) (-35.732, -13.7432) (-35.5383, -13.6938) knots 0 0 0 0 1 1 1 1
  arc A46 (-35.0676, -13.9336) -> (-35.5383, -13.6938) centre (-35.4393, -14.0813) ccw
  arc A47 (-34.8123, -15.4464) -> (-34.6491, -14.944) centre (-35.0164, -15.1024) ccw
  spline S45 degree 3 poles (-39.953, -13.7857) (-38.4112, -13.9863) (-37.2502, -13.9482) (-36.4722, -13.8582) knots 0 0 0 0 1 1 1 1
  spline S46 degree 3 poles (-37.6523, -10.2263) (-38.3346, -10.6107) (-39.2962, -11.2623) (-40.4257, -12.331) knots 0 0 0 0 1 1 1 1
  arc A48 (-32.4562, -19.2479) -> (-31.8848, -20.1803) centre (0, 0) ccw
  arc A49 (-31.9674, -20.7021) -> (-31.8848, -20.1803) centre (-32.2228, -20.3942) ccw
  spline S47 degree 3 poles (-35.5889, -15.9905) (-36.2028, -16.477) (-37.0506, -17.271) (-37.999, -18.5031) knots 0 0 0 0 1 1 1 1
  arc A50 (-35.0676, -13.9336) -> (-34.6491, -14.944) centre (0, 0) ccw
  spline S48 degree 3 poles (-37.3046, -19.866) (-35.7503, -19.823) (-34.6096, -19.6037) (-33.8552, -19.3931) knots 0 0 0 0 1 1 1 1
  arc A51 (-32.4562, -19.2479) -> (-32.9586, -19.0846) centre (-32.8002, -19.4519) ccw
  arc A52 (-34.6367, -24.2197) -> (-33.7376, -25.4571) centre (0, 0) ccw
  spline S49 degree 3 poles (-34.8123, -15.4464) (-34.9843, -15.5484) (-35.2478, -15.7204) (-35.5889, -15.9905) knots 0 0 0 0 1 1 1 1
  spline S50 degree 3 poles (-32.6493, -21.3609) (-33.1795, -21.9375) (-33.8927, -22.8543) (-34.6367, -24.2197) knots 0 0 0 0 1 1 1 1
  spline S51 degree 3 poles (-33.8552, -19.3931) (-33.4362, -19.2759) (-33.1422, -19.1638) (-32.9586, -19.0846) knots 0 0 0 0 1 1 1 1
  spline S52 degree 3 poles (-33.7376, -25.4571) (-32.2092, -25.1715) (-31.1168, -24.7765) (-30.4047, -24.4505) knots 0 0 0 0 1 1 1 1
  spline S53 degree 3 poles (-28.3353, -25.448) (-28.4673, -25.5981) (-28.6648, -25.8431) (-28.9058, -26.2054) knots 0 0 0 0 1 1 1 1
  arc A53 (-37.999, -18.5031) -> (-37.3046, -19.866) centre (0, 0) ccw
  arc A54 (-29.0455, -24.0882) -> (-28.3353, -24.9197) centre (0, 0) ccw
  spline S54 degree 3 poles (-31.9674, -20.7021) (-32.1213, -20.8297) (-32.3546, -21.0408) (-32.6493, -21.3609) knots 0 0 0 0 1 1 1 1
  spline S55 degree 3 poles (-30.4047, -24.4505) (-30.0091, -24.2691) (-29.7363, -24.1124) (-29.5673, -24.0055) knots 0 0 0 0 1 1 1 1
  arc A55 (-28.3353, -25.448) -> (-28.3353, -24.9197) centre (-28.6357, -25.1839) ccw
  arc A56 (-30.4214, -29.3399) -> (-29.3399, -30.4214) centre (0, 0) ccw
  spline S56 degree 3 poles (-29.3399, -30.4214) (-27.8749, -29.9002) (-26.8578, -29.3392) (-26.2054, -28.9058) knots 0 0 0 0 1 1 1 1
  spline S57 degree 3 poles (-28.9058, -26.2054) (-29.3392, -26.8578) (-29.9002, -27.8749) (-30.4214, -29.3399) knots 0 0 0 0 1 1 1 1
  spline S58 degree 3 poles (-24.4505, -30.4047) (-24.7765, -31.1168) (-25.1715, -32.2092) (-25.4571, -33.7376) knots 0 0 0 0 1 1 1 1
  arc A57 (-25.4571, -33.7376) -> (-24.2197, -34.6367) centre (0, 0) ccw
  arc A58 (-19.0846, -32.9586) -> (-19.2479, -32.4562) centre (-19.4519, -32.8002) ccw
  arc A59 (-29.0455, -24.0882) -> (-29.5673, -24.0055) centre (-29.3534, -24.3435) ccw
  arc A60 (-24.9197, -28.3353) -> (-24.0882, -29.0455) centre (0, 0) ccw
  spline S59 degree 3 poles (-24.0055, -29.5673) (-24.1124, -29.7363) (-24.2691, -30.0091) (-24.4505, -30.4047) knots 0 0 0 0 1 1 1 1
  spline S60 degree 3 poles (-26.2054, -28.9058) (-25.8431, -28.6648) (-25.5981, -28.4673) (-25.448, -28.3353) knots 0 0 0 0 1 1 1 1
  arc A61 (-24.9197, -28.3353) -> (-25.448, -28.3353) centre (-25.1839, -28.6357) ccw
  arc A62 (-24.0055, -29.5673) -> (-24.0882, -29.0455) centre (-24.3435, -29.3534) ccw
  spline S61 degree 3 poles (-25.448, 28.3353) (-25.5981, 28.4673) (-25.8431, 28.6648) (-26.2054, 28.9058) knots 0 0 0 0 1 1 1 1
  spline S62 degree 3 poles (-30.4047, 24.4505) (-31.1168, 24.7765) (-32.2092, 25.1715) (-33.7376, 25.4571) knots 0 0 0 0 1 1 1 1
  spline S63 degree 3 poles (-24.4505, 30.4047) (-24.2691, 30.0091) (-24.1124, 29.7363) (-24.0055, 29.5673) knots 0 0 0 0 1 1 1 1
  arc A63 (-29.5673, 24.0055) -> (-29.0455, 24.0882) centre (-29.3534, 24.3435) ccw
  arc A64 (-28.3353, 24.9197) -> (-28.3353, 25.448) centre (-28.6357, 25.1839) ccw
  arc A65 (-33.7376, 25.4571) -> (-34.6367, 24.2197) centre (0, 0) ccw
  arc A66 (-29.3399, 30.4214) -> (-30.4214, 29.3399) centre (0, 0) ccw
  arc A67 (-25.448, 28.3353) -> (-24.9197, 28.3353) centre (-25.1839, 28.6357) ccw
  arc A68 (-28.3353, 24.9197) -> (-29.0455, 24.0882) centre (0, 0) ccw
  spline S64 degree 3 poles (-28.9058, 26.2054) (-28.6648, 25.8431) (-28.4673, 25.5981) (-28.3353, 25.448) knots 0 0 0 0 1 1 1 1
  spline S65 degree 3 poles (-26.2054, 28.9058) (-26.8578, 29.3392) (-27.8749, 29.9002) (-29.3399, 30.4214) knots 0 0 0 0 1 1 1 1
  spline S66 degree 3 poles (-30.4214, 29.3399) (-29.9002, 27.8749) (-29.3392, 26.8578) (-28.9058, 26.2054) knots 0 0 0 0 1 1 1 1
  spline S67 degree 3 poles (-29.5673, 24.0055) (-29.7363, 24.1124) (-30.0091, 24.2691) (-30.4047, 24.4505) knots 0 0 0 0 1 1 1 1
  arc A69 (8.2763, -36.8156) -> (9.3397, -36.5603) centre (0, 0) ccw
  spline S68 degree 3 poles (7.9821, -38.191) (8.0001, -37.7562) (7.9843, -37.442) (7.9658, -37.243) knots 0 0 0 0 1 1 1 1
  spline S69 degree 3 poles (7.3659, -41.6177) (7.8053, -40.1262) (7.9493, -38.9736) (7.9821, -38.191) knots 0 0 0 0 1 1 1 1
  arc A70 (8.2763, -36.8156) -> (7.9658, -37.243) centre (8.364, -37.2058) ccw
  arc A71 (12.331, -40.4257) -> (13.7857, -39.953) centre (0, 0) ccw
  spline S70 degree 3 poles (9.8104, -36.8001) (9.8842, -36.9859) (10.0128, -37.273) (10.2263, -37.6523) knots 0 0 0 0 1 1 1 1
  spline S71 degree 3 poles (10.2263, -37.6523) (10.6107, -38.3346) (11.2623, -39.2962) (12.331, -40.4257) knots 0 0 0 0 1 1 1 1
  arc A72 (9.8104, -36.8001) -> (9.3397, -36.5603) centre (9.4387, -36.9478) ccw
  spline S72 degree 3 poles (13.7857, -39.953) (13.9863, -38.4112) (13.9482, -37.2502) (13.8582, -36.4722) knots 0 0 0 0 1 1 1 1
  arc A73 (13.9336, -35.0676) -> (14.944, -34.6491) centre (0, 0) ccw
  spline S73 degree 3 poles (15.4464, -34.8123) (15.5484, -34.9843) (15.7204, -35.2478) (15.9905, -35.5889) knots 0 0 0 0 1 1 1 1
  arc A74 (13.9336, -35.0676) -> (13.6938, -35.5383) centre (14.0813, -35.4393) ccw
  spline S74 degree 3 poles (13.8582, -36.4722) (13.808, -36.0399) (13.7432, -35.732) (13.6938, -35.5383) knots 0 0 0 0 1 1 1 1
  spline S75 degree 3 poles (15.9905, -35.5889) (16.477, -36.2028) (17.271, -37.0506) (18.5031, -37.999) knots 0 0 0 0 1 1 1 1
  arc A75 (18.5031, -37.999) -> (19.866, -37.3046) centre (0, 0) ccw
  spline S76 degree 3 poles (20.7021, -31.9674) (20.8297, -32.1213) (21.0408, -32.3546) (21.3609, -32.6493) knots 0 0 0 0 1 1 1 1
  arc A76 (24.0882, -29.0455) -> (24.0055, -29.5673) centre (24.3435, -29.3534) ccw
  arc A77 (19.2479, -32.4562) -> (19.0846, -32.9586) centre (19.4519, -32.8002) ccw
  spline S77 degree 3 poles (19.3931, -33.8552) (19.2759, -33.4362) (19.1638, -33.1422) (19.0846, -32.9586) knots 0 0 0 0 1 1 1 1
  arc A78 (15.4464, -34.8123) -> (14.944, -34.6491) centre (15.1024, -35.0164) ccw
  spline S78 degree 3 poles (19.866, -37.3046) (19.823, -35.7503) (19.6037, -34.6096) (19.3931, -33.8552) knots 0 0 0 0 1 1 1 1
  arc A79 (20.7021, -31.9674) -> (20.1803, -31.8848) centre (20.3942, -32.2228) ccw
  arc A80 (19.2479, -32.4562) -> (20.1803, -31.8848) centre (0, 0) ccw
  spline S79 degree 3 poles (24.4505, -30.4047) (24.2691, -30.0091) (24.1124, -29.7363) (24.0055, -29.5673) knots 0 0 0 0 1 1 1 1
  spline S80 degree 3 poles (21.3609, -32.6493) (21.9375, -33.1795) (22.8543, -33.8927) (24.2197, -34.6367) knots 0 0 0 0 1 1 1 1
  arc A81 (24.2197, -34.6367) -> (25.4571, -33.7376) centre (0, 0) ccw
  arc A82 (24.0882, -29.0455) -> (24.9197, -28.3353) centre (0, 0) ccw
  arc A83 (25.448, -28.3353) -> (24.9197, -28.3353) centre (25.1839, -28.6357) ccw
  arc A84 (29.3399, -30.4214) -> (30.4214, -29.3399) centre (0, 0) ccw
  spline S81 degree 3 poles (26.2054, -28.9058) (26.8578, -29.3392) (27.8749, -29.9002) (29.3399, -30.4214) knots 0 0 0 0 1 1 1 1
  spline S82 degree 3 poles (25.448, -28.3353) (25.5981, -28.4673) (25.8431, -28.6648) (26.2054, -28.9058) knots 0 0 0 0 1 1 1 1
  spline S83 degree 3 poles (25.4571, -33.7376) (25.1715, -32.2092) (24.7765, -31.1168) (24.4505, -30.4047) knots 0 0 0 0 1 1 1 1
  spline S84 degree 3 poles (28.9058, -26.2054) (28.6648, -25.8431) (28.4673, -25.5981) (28.3353, -25.448) knots 0 0 0 0 1 1 1 1
  arc A85 (28.3353, -24.9197) -> (28.3353, -25.448) centre (28.6357, -25.1839) ccw
  arc A86 (29.5673, -24.0055) -> (29.0455, -24.0882) centre (29.3534, -24.3435) ccw
  spline S85 degree 3 poles (29.5673, -24.0055) (29.7363, -24.1124) (30.0091, -24.2691) (30.4047, -24.4505) knots 0 0 0 0 1 1 1 1
  arc A87 (33.7376, -25.4571) -> (34.6367, -24.2197) centre (0, 0) ccw
  arc A88 (28.3353, -24.9197) -> (29.0455, -24.0882) centre (0, 0) ccw
  spline S86 degree 3 poles (30.4214, -29.3399) (29.9002, -27.8749) (29.3392, -26.8578) (28.9058, -26.2054) knots 0 0 0 0 1 1 1 1
  arc A89 (-34.6491, 14.944) -> (-35.0676, 13.9336) centre (0, 0) ccw
  spline S87 degree 3 poles (-35.5383, 13.6938) (-35.732, 13.7432) (-36.0399, 13.808) (-36.4722, 13.8582) knots 0 0 0 0 1 1 1 1
  spline S88 degree 3 poles (30.4047, -24.4505) (31.1168, -24.7765) (32.2092, -25.1715) (33.7376, -25.4571) knots 0 0 0 0 1 1 1 1
  spline S89 degree 3 poles (-35.5889, 15.9905) (-35.2478, 15.7204) (-34.9843, 15.5484) (-34.8123, 15.4464) knots 0 0 0 0 1 1 1 1
  arc A90 (-35.5383, 13.6938) -> (-35.0676, 13.9336) centre (-35.4393, 14.0813) ccw
  spline S90 degree 3 poles (-41.857, 5.8552) (-40.5743, 4.9764) (-39.5225, 4.4833) (-38.7884, 4.2102) knots 0 0 0 0 1 1 1 1
  spline S91 degree 3 poles (-34.6367, 24.2197) (-33.8927, 22.8543) (-33.1795, 21.9375) (-32.6493, 21.3609) knots 0 0 0 0 1 1 1 1
  arc A91 (-36.5603, 9.3397) -> (-36.8156, 8.2763) centre (0, 0) ccw
  spline S92 degree 3 poles (-32.9586, 19.0846) (-33.1422, 19.1638) (-33.4362, 19.2759) (-33.8552, 19.3931) knots 0 0 0 0 1 1 1 1
  arc A92 (-31.8848, 20.1803) -> (-32.4562, 19.2479) centre (0, 0) ccw
  spline S93 degree 3 poles (-37.243, 7.9658) (-37.442, 7.9843) (-37.7562, 8.0001) (-38.191, 7.9821) knots 0 0 0 0 1 1 1 1
  arc A93 (-31.8848, 20.1803) -> (-31.9674, 20.7021) centre (-32.2228, 20.3942) ccw
  spline S94 degree 3 poles (-32.6493, 21.3609) (-32.3546, 21.0408) (-32.1213, 20.8297) (-31.9674, 20.7021) knots 0 0 0 0 1 1 1 1
  spline S95 degree 3 poles (-33.8552, 19.3931) (-34.6096, 19.6037) (-35.7503, 19.823) (-37.3046, 19.866) knots 0 0 0 0 1 1 1 1
  arc A94 (-37.243, 7.9658) -> (-36.8156, 8.2763) centre (-37.2058, 8.364) ccw
  arc A95 (-37.3046, 19.866) -> (-37.999, 18.5031) centre (0, 0) ccw
  arc A96 (-32.9586, 19.0846) -> (-32.4562, 19.2479) centre (-32.8002, 19.4519) ccw
  spline S96 degree 3 poles (-37.999, 18.5031) (-37.0506, 17.271) (-36.2028, 16.477) (-35.5889, 15.9905) knots 0 0 0 0 1 1 1 1
  spline S97 degree 3 poles (-37.6523, 10.2263) (-37.273, 10.0128) (-36.9859, 9.8842) (-36.8001, 9.8104) knots 0 0 0 0 1 1 1 1
  spline S98 degree 3 poles (-40.4257, 12.331) (-39.2962, 11.2623) (-38.3346, 10.6107) (-37.6523, 10.2263) knots 0 0 0 0 1 1 1 1
  arc A97 (-41.6177, 7.3659) -> (-41.857, 5.8552) centre (0, 0) ccw
  spline S99 degree 3 poles (-36.4722, 13.8582) (-37.2502, 13.9482) (-38.4112, 13.9863) (-39.953, 13.7857) knots 0 0 0 0 1 1 1 1
  arc A98 (-36.5603, 9.3397) -> (-36.8001, 9.8104) centre (-36.9478, 9.4387) ccw
  arc A99 (-39.953, 13.7857) -> (-40.4257, 12.331) centre (0, 0) ccw
  arc A100 (-34.6491, 14.944) -> (-34.8123, 15.4464) centre (-35.0164, 15.1024) ccw
  spline S100 degree 3 poles (-38.191, 7.9821) (-38.9736, 7.9493) (-40.1262, 7.8053) (-41.6177, 7.3659) knots 0 0 0 0 1 1 1 1
  arc A101 (38.0306, -2.0416) -> (37.657, -2.4152) centre (38.0562, -2.4408) ccw
  spline S101 degree 3 poles (42.2576, 0.7648) (40.8532, 1.4321) (39.7373, 1.7546) (38.9695, 1.9094) knots 0 0 0 0 1 1 1 1
  spline S102 degree 3 poles (38.9695, -1.9094) (39.7373, -1.7546) (40.8532, -1.4321) (42.2576, -0.7648) knots 0 0 0 0 1 1 1 1
  arc A102 (42.2576, -0.7648) -> (42.2576, 0.7648) centre (0, 0) ccw
  spline S103 degree 3 poles (38.0306, -2.0416) (38.23, -2.0288) (38.5429, -1.9952) (38.9695, -1.9094) knots 0 0 0 0 1 1 1 1
  arc A103 (37.8817, 3.9328) -> (37.5712, 3.5054) centre (37.9695, 3.5426) ccw
  spline S104 degree 3 poles (38.9695, 1.9094) (38.5429, 1.9952) (38.23, 2.0288) (38.0306, 2.0416) knots 0 0 0 0 1 1 1 1
  spline S105 degree 3 poles (38.7884, 4.2102) (39.5225, 4.4833) (40.5743, 4.9764) (41.857, 5.8552) knots 0 0 0 0 1 1 1 1
  spline S106 degree 3 poles (37.8817, 3.9328) (38.0767, 3.9767) (38.3805, 4.0588) (38.7884, 4.2102) knots 0 0 0 0 1 1 1 1
  arc A104 (37.657, 2.4152) -> (38.0306, 2.0416) centre (38.0562, 2.4408) ccw
  arc A105 (36.8156, 8.2763) -> (36.5603, 9.3397) centre (0, 0) ccw
  arc A106 (40.4257, 12.331) -> (39.953, 13.7857) centre (0, 0) ccw
  arc A107 (37.657, 2.4152) -> (37.5712, 3.5054) centre (0, 0) ccw
  arc A108 (36.8001, 9.8104) -> (36.5603, 9.3397) centre (36.9478, 9.4387) ccw
  arc A109 (41.857, 5.8552) -> (41.6177, 7.3659) centre (0, 0) ccw
  spline S107 degree 3 poles (38.191, 7.9821) (37.7562, 8.0001) (37.442, 7.9843) (37.243, 7.9658) knots 0 0 0 0 1 1 1 1
  spline S108 degree 3 poles (41.6177, 7.3659) (40.1262, 7.8053) (38.9736, 7.9493) (38.191, 7.9821) knots 0 0 0 0 1 1 1 1
  spline S109 degree 3 poles (36.8001, 9.8104) (36.9859, 9.8842) (37.273, 10.0128) (37.6523, 10.2263) knots 0 0 0 0 1 1 1 1
  arc A110 (36.8156, 8.2763) -> (37.243, 7.9658) centre (37.2058, 8.364) ccw
  spline S110 degree 3 poles (35.5889, 15.9905) (36.2028, 16.477) (37.0506, 17.271) (37.999, 18.5031) knots 0 0 0 0 1 1 1 1
  arc A111 (35.0676, 13.9336) -> (34.6491, 14.944) centre (0, 0) ccw
  arc A112 (34.8123, 15.4464) -> (34.6491, 14.944) centre (35.0164, 15.1024) ccw
  arc A113 (35.0676, 13.9336) -> (35.5383, 13.6938) centre (35.4393, 14.0813) ccw
  spline S111 degree 3 poles (36.4722, 13.8582) (36.0399, 13.808) (35.732, 13.7432) (35.5383, 13.6938) knots 0 0 0 0 1 1 1 1
  arc A114 (37.999, 18.5031) -> (37.3046, 19.866) centre (0, 0) ccw
  spline S112 degree 3 poles (37.6523, 10.2263) (38.3346, 10.6107) (39.2962, 11.2623) (40.4257, 12.331) knots 0 0 0 0 1 1 1 1
  spline S113 degree 3 poles (32.6493, 21.3609) (33.1795, 21.9375) (33.8927, 22.8543) (34.6367, 24.2197) knots 0 0 0 0 1 1 1 1
  spline S114 degree 3 poles (33.8552, 19.3931) (33.4362, 19.2759) (33.1422, 19.1638) (32.9586, 19.0846) knots 0 0 0 0 1 1 1 1
  spline S115 degree 3 poles (39.953, 13.7857) (38.4112, 13.9863) (37.2502, 13.9482) (36.4722, 13.8582) knots 0 0 0 0 1 1 1 1
  spline S116 degree 3 poles (34.8123, 15.4464) (34.9843, 15.5484) (35.2478, 15.7204) (35.5889, 15.9905) knots 0 0 0 0 1 1 1 1
  spline S117 degree 3 poles (37.3046, 19.866) (35.7503, 19.823) (34.6096, 19.6037) (33.8552, 19.3931) knots 0 0 0 0 1 1 1 1
  arc A115 (34.6367, 24.2197) -> (33.7376, 25.4571) centre (0, 0) ccw
  arc A116 (31.9674, 20.7021) -> (31.8848, 20.1803) centre (32.2228, 20.3942) ccw
  spline S118 degree 3 poles (31.9674, 20.7021) (32.1213, 20.8297) (32.3546, 21.0408) (32.6493, 21.3609) knots 0 0 0 0 1 1 1 1
  arc A117 (32.4562, 19.2479) -> (32.9586, 19.0846) centre (32.8002, 19.4519) ccw
  spline S119 degree 3 poles (30.4047, 24.4505) (30.0091, 24.2691) (29.7363, 24.1124) (29.5673, 24.0055) knots 0 0 0 0 1 1 1 1
  arc A118 (32.4562, 19.2479) -> (31.8848, 20.1803) centre (0, 0) ccw
  arc A119 (24.9197, 28.3353) -> (24.0882, 29.0455) centre (0, 0) ccw
  arc A120 (30.4214, 29.3399) -> (29.3399, 30.4214) centre (0, 0) ccw
  spline S120 degree 3 poles (24.4505, 30.4047) (24.7765, 31.1168) (25.1715, 32.2092) (25.4571, 33.7376) knots 0 0 0 0 1 1 1 1
  spline S121 degree 3 poles (33.7376, 25.4571) (32.2092, 25.1715) (31.1168, 24.7765) (30.4047, 24.4505) knots 0 0 0 0 1 1 1 1
  arc A121 (24.0055, 29.5673) -> (24.0882, 29.0455) centre (24.3435, 29.3534) ccw
  arc A122 (24.9197, 28.3353) -> (25.448, 28.3353) centre (25.1839, 28.6357) ccw
  arc A123 (20.1803, 31.8848) -> (19.2479, 32.4562) centre (0, 0) ccw
  spline S122 degree 3 poles (28.9058, 26.2054) (29.3392, 26.8578) (29.9002, 27.8749) (30.4214, 29.3399) knots 0 0 0 0 1 1 1 1
  spline S123 degree 3 poles (29.3399, 30.4214) (27.8749, 29.9002) (26.8578, 29.3392) (26.2054, 28.9058) knots 0 0 0 0 1 1 1 1
  arc A124 (28.3353, 25.448) -> (28.3353, 24.9197) centre (28.6357, 25.1839) ccw
  spline S124 degree 3 poles (26.2054, 28.9058) (25.8431, 28.6648) (25.5981, 28.4673) (25.448, 28.3353) knots 0 0 0 0 1 1 1 1
  spline S125 degree 3 poles (24.0055, 29.5673) (24.1124, 29.7363) (24.2691, 30.0091) (24.4505, 30.4047) knots 0 0 0 0 1 1 1 1
  spline S126 degree 3 poles (28.3353, 25.448) (28.4673, 25.5981) (28.6648, 25.8431) (28.9058, 26.2054) knots 0 0 0 0 1 1 1 1
  arc A125 (29.0455, 24.0882) -> (29.5673, 24.0055) centre (29.3534, 24.3435) ccw
  arc A126 (19.0846, 32.9586) -> (19.2479, 32.4562) centre (19.4519, 32.8002) ccw
  spline S127 degree 3 poles (21.3609, 32.6493) (21.0408, 32.3546) (20.8297, 32.1213) (20.7021, 31.9674) knots 0 0 0 0 1 1 1 1
  arc A127 (29.0455, 24.0882) -> (28.3353, 24.9197) centre (0, 0) ccw
  arc A128 (25.4571, 33.7376) -> (24.2197, 34.6367) centre (0, 0) ccw
  arc A129 (20.1803, 31.8848) -> (20.7021, 31.9674) centre (20.3942, 32.2228) ccw
  spline S128 degree 3 poles (24.2197, 34.6367) (22.8543, 33.8927) (21.9375, 33.1795) (21.3609, 32.6493) knots 0 0 0 0 1 1 1 1
  spline S129 degree 3 poles (19.0846, 32.9586) (19.1638, 33.1422) (19.2759, 33.4362) (19.3931, 33.8552) knots 0 0 0 0 1 1 1 1
  spline S130 degree 3 poles (19.3931, 33.8552) (19.6037, 34.6096) (19.823, 35.7503) (19.866, 37.3046) knots 0 0 0 0 1 1 1 1
  arc A130 (14.944, 34.6491) -> (13.9336, 35.0676) centre (0, 0) ccw
  arc A131 (13.6938, 35.5383) -> (13.9336, 35.0676) centre (14.0813, 35.4393) ccw
  spline S131 degree 3 poles (13.6938, 35.5383) (13.7432, 35.732) (13.808, 36.0399) (13.8582, 36.4722) knots 0 0 0 0 1 1 1 1
  arc A132 (14.944, 34.6491) -> (15.4464, 34.8123) centre (15.1024, 35.0164) ccw
  arc A133 (19.866, 37.3046) -> (18.5031, 37.999) centre (0, 0) ccw
  spline S132 degree 3 poles (18.5031, 37.999) (17.271, 37.0506) (16.477, 36.2028) (15.9905, 35.5889) knots 0 0 0 0 1 1 1 1
  spline S133 degree 3 poles (15.9905, 35.5889) (15.7204, 35.2478) (15.5484, 34.9843) (15.4464, 34.8123) knots 0 0 0 0 1 1 1 1
  arc A134 (9.3397, 36.5603) -> (9.8104, 36.8001) centre (9.4387, 36.9478) ccw
  arc A135 (7.3659, 41.6177) -> (5.8552, 41.857) centre (0, 0) ccw
  spline S134 degree 3 poles (10.2263, 37.6523) (10.0128, 37.273) (9.8842, 36.9859) (9.8104, 36.8001) knots 0 0 0 0 1 1 1 1
  spline S135 degree 3 poles (1.9094, 38.9695) (1.7546, 39.7373) (1.4321, 40.8532) (0.7648, 42.2576) knots 0 0 0 0 1 1 1 1
  arc A136 (0.7648, 42.2576) -> (-0.7648, 42.2576) centre (0, 0) ccw
  spline S136 degree 3 poles (2.0416, 38.0306) (2.0288, 38.23) (1.9952, 38.5429) (1.9094, 38.9695) knots 0 0 0 0 1 1 1 1
  spline S137 degree 3 poles (12.331, 40.4257) (11.2623, 39.2962) (10.6107, 38.3346) (10.2263, 37.6523) knots 0 0 0 0 1 1 1 1
  arc A137 (3.5054, 37.5712) -> (2.4152, 37.657) centre (0, 0) ccw
  arc A138 (7.9658, 37.243) -> (8.2763, 36.8156) centre (8.364, 37.2058) ccw
  spline S138 degree 3 poles (4.2102, 38.7884) (4.0588, 38.3805) (3.9767, 38.0767) (3.9328, 37.8817) knots 0 0 0 0 1 1 1 1
  arc A139 (-5.8552, 41.857) -> (-7.3659, 41.6177) centre (0, 0) ccw
  spline S139 degree 3 poles (-3.9328, 37.8817) (-3.9767, 38.0767) (-4.0588, 38.3805) (-4.2102, 38.7884) knots 0 0 0 0 1 1 1 1
  arc A140 (13.7857, 39.953) -> (12.331, 40.4257) centre (0, 0) ccw
  spline S140 degree 3 poles (7.9658, 37.243) (7.9843, 37.442) (8.0001, 37.7562) (7.9821, 38.191) knots 0 0 0 0 1 1 1 1
  arc A141 (3.5054, 37.5712) -> (3.9328, 37.8817) centre (3.5426, 37.9695) ccw
  arc A142 (2.0416, 38.0306) -> (2.4152, 37.657) centre (2.4408, 38.0562) ccw
  spline S141 degree 3 poles (5.8552, 41.857) (4.9764, 40.5743) (4.4833, 39.5225) (4.2102, 38.7884) knots 0 0 0 0 1 1 1 1
  arc A143 (9.3397, 36.5603) -> (8.2763, 36.8156) centre (0, 0) ccw
  spline S142 degree 3 poles (13.8582, 36.4722) (13.9482, 37.2502) (13.9863, 38.4112) (13.7857, 39.953) knots 0 0 0 0 1 1 1 1
  spline S143 degree 3 poles (7.9821, 38.191) (7.9493, 38.9736) (7.8053, 40.1262) (7.3659, 41.6177) knots 0 0 0 0 1 1 1 1
  spline S144 degree 3 poles (-7.3659, 41.6177) (-7.8053, 40.1262) (-7.9493, 38.9736) (-7.9821, 38.191) knots 0 0 0 0 1 1 1 1
  arc A144 (-8.2763, 36.8156) -> (-7.9658, 37.243) centre (-8.364, 37.2058) ccw
  arc A145 (-12.331, 40.4257) -> (-13.7857, 39.953) centre (0, 0) ccw
  arc A146 (-2.4152, 37.657) -> (-2.0416, 38.0306) centre (-2.4408, 38.0562) ccw
  spline S145 degree 3 poles (-9.8104, 36.8001) (-9.8842, 36.9859) (-10.0128, 37.273) (-10.2263, 37.6523) knots 0 0 0 0 1 1 1 1
  arc A147 (-13.9336, 35.0676) -> (-13.6938, 35.5383) centre (-14.0813, 35.4393) ccw
  arc A148 (-3.9328, 37.8817) -> (-3.5054, 37.5712) centre (-3.5426, 37.9695) ccw
  spline S146 degree 3 poles (-0.7648, 42.2576) (-1.4321, 40.8532) (-1.7546, 39.7373) (-1.9094, 38.9695) knots 0 0 0 0 1 1 1 1
  arc A149 (-2.4152, 37.657) -> (-3.5054, 37.5712) centre (0, 0) ccw
  spline S147 degree 3 poles (-4.2102, 38.7884) (-4.4833, 39.5225) (-4.9764, 40.5743) (-5.8552, 41.857) knots 0 0 0 0 1 1 1 1
  spline S148 degree 3 poles (-15.4464, 34.8123) (-15.5484, 34.9843) (-15.7204, 35.2478) (-15.9905, 35.5889) knots 0 0 0 0 1 1 1 1